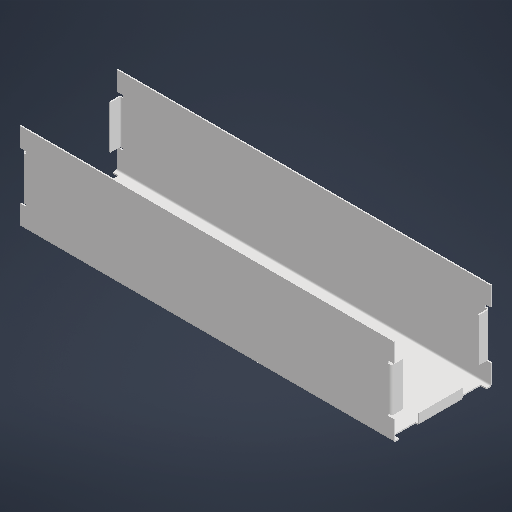
# Autodesk Inventor part: Bottom
Saved by Autodesk Inventor 2026.1 (Build 301233020, 233B)
## iProperties
Created: 2025-11-02
Part Number: Bottom
Material: Generic
Document SubType Name: Sheet Metal
Designer: 박정현
Density: 1 g/cm^3
Sheet Metal Rule: Default
Appearance: Default
Author: 박정현
Autodesk Inventor part; units mm, degrees
ref_plane "YZ Plane" through (0, 0, 0) normal (1, 0, 0) x (0, 1, 0)
ref_plane "XZ Plane" through (0, 0, 0) normal (0, 1, 0) x (-1, 0, 0)
ref_plane "XY Plane" through (0, 0, 0) normal (0, 0, 1) x (1, 0, 0)
sketch "Sketch1" plane through (0, 0, 0) normal (0, 1, 0) x (-1, 0, 0)
  line L0 (208, -50) -> (-208, -50)
  line L1 (-208, -50) -> (-208, 50)
  line L2 (-208, 50) -> (208, 50)
  line L3 (208, 50) -> (208, -50)
  line L4 (215, 50) -> (-215, 50)
  line L5 (-215, 50) -> (-215, 78)
  line L6 (-215, 78) -> (215, 78)
  line L7 (215, 78) -> (215, 50)
  line L8 (215, -50) -> (-215, -50)
  line L9 (-215, -50) -> (-215, -78)
  line L10 (-215, -78) -> (215, -78)
  line L11 (215, -78) -> (215, -50)
  line L12 (208, 78) -> (-208, 78)
  line L13 (-208, 78) -> (-208, 133)
  line L14 (-208, 133) -> (208, 133)
  line L15 (208, 133) -> (208, 78)
  line L16 (215, 133) -> (-215, 133)
  line L17 (-215, 133) -> (-215, 155)
  line L18 (-215, 155) -> (215, 155)
  line L19 (215, 155) -> (215, 133)
  line L20 (208, -78) -> (-208, -78)
  line L21 (-208, -78) -> (-208, -133)
  line L22 (-208, -133) -> (208, -133)
  line L23 (208, -133) -> (208, -78)
  line L24 (215, -133) -> (-215, -133)
  line L25 (-215, -133) -> (-215, -155)
  line L26 (-215, -155) -> (215, -155)
  line L27 (215, -155) -> (215, -133)
  line L28 (208, -25) -> (213, -25)
  line L29 (213, -25) -> (213, 25)
  line L30 (213, 25) -> (208, 25)
  line L31 (208, 25) -> (208, -25)
  line L32 (213, -25) -> (223, -25)
  line L33 (223, -25) -> (223, 25)
  line L34 (223, 25) -> (213, 25)
  line L35 (213, 25) -> (213, -25)
  line L36 (-208, -25) -> (-213, -25)
  line L37 (-213, -25) -> (-213, 25)
  line L38 (-213, 25) -> (-208, 25)
  line L39 (-208, 25) -> (-208, -25)
  line L40 (-213, -25) -> (-223, -25)
  line L41 (-223, -25) -> (-223, 25)
  line L42 (-223, 25) -> (-213, 25)
  line L43 (-213, 25) -> (-213, -25)
  line L44 (208, 80) -> (213, 80)
  line L45 (213, 80) -> (213, 130)
  line L46 (213, 130) -> (208, 130)
  line L47 (208, 130) -> (208, 80)
  line L48 (213, 80) -> (223, 80)
  line L49 (223, 80) -> (223, 130)
  line L50 (223, 130) -> (213, 130)
  line L51 (213, 130) -> (213, 80)
  line L52 (-208, 80) -> (-213, 80)
  line L53 (-213, 80) -> (-213, 130)
  line L54 (-213, 130) -> (-208, 130)
  line L55 (-208, 130) -> (-208, 80)
  line L56 (-213, 80) -> (-223, 80)
  line L57 (-223, 80) -> (-223, 130)
  line L58 (-223, 130) -> (-213, 130)
  line L59 (-213, 130) -> (-213, 80)
  line L60 (208, -130) -> (213, -130)
  line L61 (213, -130) -> (213, -80)
  line L62 (213, -80) -> (208, -80)
  line L63 (208, -80) -> (208, -130)
  line L64 (213, -130) -> (223, -130)
  line L65 (223, -130) -> (223, -80)
  line L66 (223, -80) -> (213, -80)
  line L67 (213, -80) -> (213, -130)
  line L68 (-208, -130) -> (-213, -130)
  line L69 (-213, -130) -> (-213, -80)
  line L70 (-213, -80) -> (-208, -80)
  line L71 (-208, -80) -> (-208, -130)
  line L72 (-213, -130) -> (-223, -130)
  line L73 (-223, -130) -> (-223, -80)
  line L74 (-223, -80) -> (-213, -80)
  line L75 (-213, -80) -> (-213, -130)
  line L76 (208, 50) -> (-208, -50) construction
  line L77 (-208, 50) -> (208, -50) construction
  line L78 (215, -57) -> (-215, -57) construction
  line L79 (215, 57) -> (-215, 57) construction
  point P0 (0, 0)
  point P1 (208, 0)
  point P2 (-208, 0)
  point P3 (208, 25)
  point P4 (208, 50)
  point P5 (208, 133)
  point P6 (-208, 133)
  point P7 (-208, 130)
  point P8 (-208, 78)
  point P9 (-208, 50)
  point P10 (-208, 25)
  point P11 (-208, -50)
  point P12 (-208, -78)
  point P13 (-208, -133)
  point P14 (208, -133)
  point P15 (208, -50)
  dimension "d0" = 430
  dimension "d1" = 7
  dimension "d3" = 100
  dimension "d4" = 50
  dimension "d5" = 50
  dimension "d7" = 5
  dimension "d8" = 50
  dimension "d9" = 50
  dimension "d10" = 10
  dimension "d11" = 10
  dimension "d12" = 105
  dimension "d13" = 105
  dimension "d14" = 28
  dimension "d15" = 28
  dimension "d16" = 25
  dimension "d17" = 25
  dimension "d18" = 22
  dimension "d19" = 22
  dimension "d57" = 7
  dimension "d58" = 7
  dimension "d71" = 7
  dimension "d72" = 5
  constraints: 160 end point, 39 point on line, 38 parallel, 21 perpendicular, 19 horizontal, 6 midpoint, 5 collinear, 1 other
  measures "d0" distance of L17.end L18.end
  measures "d1" distance between parallel lines of L15 L19
  measures "d3" distance between parallel lines of L0 L2
  measures "d4" distance of L32.end L33.end
  measures "d5" distance of L40.end L41.end
  measures "d7" distance between parallel lines of L13 L53
  measures "d8" distance of L48.end L49.end
  measures "d9" distance of L64.end L65.end
  measures "d10" distance of L33.end L34.end
  measures "d11" distance of L41.end L42.end
  measures "d12" distance between parallel lines of L4 L18
  measures "d13" distance between parallel lines of L26 L8
  measures "d14" distance between parallel lines of L8 L10
  measures "d15" distance between parallel lines of L4 L6
  measures "d16" distance between parallel lines of L64 L26
  measures "d17" distance between parallel lines of L50 L18
  measures "d18" distance between parallel lines of L18 L16
  measures "d19" distance between parallel lines of L26 L24
  measures "d57" distance between parallel lines of L8 L78
  measures "d58" distance between parallel lines of L2 L79
  measures "d71" distance between parallel lines of L17 L13
  measures "d72" distance between parallel lines of L15 L45
extrude "Plate1" add sketch "Sketch1" against normal blind 1.5
fold "Fold1" angle 90 bend radius 1.5 thickness 1.5 k factor 0.44 line from (-213, 0, -80) to (-213, 0, -130) line at bend end moving side (-1, 0, 0) folds toward (0, 1, 0)
fold "Fold2" angle 90 bend radius 1.5 thickness 1.5 k factor 0.44 line from (-213, 0, -25) to (-213, 0, 25) line at bend end moving side (-1, 0, 0) folds toward (0, 1, 0)
fold "Fold3" angle 90 bend radius 1.5 thickness 1.5 k factor 0.44 line from (-213, 0, 130) to (-213, 0, 80) line at bend end moving side (-1, 0, 0) folds toward (0, 1, 0)
fold "Fold4" angle 90 bend radius 1.5 thickness 1.5 k factor 0.44 line from (213, 0, -80) to (213, 0, -130) line at bend end moving side (1, 0, 0) folds toward (0, 1, 0)
fold "Fold5" angle 90 bend radius 1.5 thickness 1.5 k factor 0.44 line from (213, 0, 25) to (213, 0, -25) line at bend end moving side (1, 0, 0) folds toward (0, 1, 0)
fold "Fold6" angle 90 bend radius 1.5 thickness 1.5 k factor 0.44 line from (213, 0, 80) to (213, 0, 130) line at bend end moving side (1, 0, 0) folds toward (0, 1, 0)
fold "Fold7" angle 90 bend radius 1.5 thickness 1.5 k factor 0.44 line from (-215, 0, -57) to (215, 0, -57) line at bend end moving side (0, 0, -1) folds toward (0, 1, 0)
fold "Fold8" angle 90 bend radius 1.5 thickness 1.5 k factor 0.44 line from (-215, 0, 57) to (215, 0, 57) line at bend end moving side (0, 0, 1) folds toward (0, 1, 0)
equation "\"d5\" = d4"
equation "\"d8\" = d4"
equation "\"d9\" = d4"
equation "\"d11\" = d10"
equation "\"BendRadius\" = Thickness"
equation "\"BendReliefWidth\" = Thickness"
equation "\"BendReliefDepth\" = 0.5 * Thickness"
equation "\"CornerReliefSize\" = 4 * Thickness"
equation "\"MinimumRemnant\" = 2 * Thickness"
equation "\"TransitionRadius\" = BendRadius"
equation "\"JacobiRadiusSize\" = BendRadius"
equation "\"GapSize\" = Thickness"
equation "\"Thickness\" = 1.5"
body "Solid1"
